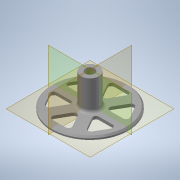
# Autodesk Inventor part: Wiel hout+spacer
Saved by Autodesk Inventor 2021 (Build 250183000, 183)
## iProperties
Manager: PJ / DCS
Company: Emmaüs Bovenbouw Aalter
Created: 2021-01-10
Part Number: Wiel hout+spacer
Material: S235
Catalog Web Link: http://emmausbovenbouw.op-weg.be/
Vendor: Emmaüsinstituut Bovenbouw Aalter
Document SubType Name: Modeling
Designer: Antho
Engineer: Declercq St.
Manufacturer: Standard
Standards Organization: Custom
Density: 7.86 g/cm^3
Appearance: Steel
Title: Algemene titel
Subject: Specifieke titel
Author: Antho
Keywords: Ruwe Ø xxxxx
Comments: Opmerking
Autodesk Inventor part; units mm, degrees
sketch "Sketch1" plane through (0, 0, 0) normal (0, 0, 1) x (1, 0, 0)
  line L0 (0, 2.8582) -> (0, -2.8582) construction
  line L1 (-5.7775, 0) -> (5.7775, 0) construction
  circle A0 centre (0, 0) radius 25.629
  circle A1 centre (0, 0) radius 4
  line L2 (0, 4) -> (0, 7)
  line L3 (0, 7) -> (0, 21)
  line L4 (0, 21) -> (5, 21)
  line L5 (5, 21) -> (8, 21)
  line L6 (8, 21) -> (0, 7)
  line L7 (0, 21) -> (-8, 21)
  line L8 (-8, 21) -> (0, 7)
  line L9 (0, -4) -> (0, -7)
  line L10 (0, -7) -> (0, -21)
  line L11 (0, -21) -> (8, -21)
  line L12 (8, -21) -> (0, -7)
  line L13 (0, -21) -> (-8, -21)
  line L14 (-8, -21) -> (0, -7)
  line L15 (0, 0) -> (2.5981, 1.5)
  line L16 (0, 0) -> (3, 0) construction
  line L17 (2.5981, 1.5) -> (3.4641, 2)
  line L18 (3.4641, 2) -> (6.0622, 3.5)
  line L19 (6.0622, 3.5) -> (18.1865, 10.5)
  line L20 (18.1865, 10.5) -> (14.1865, 17.4282)
  line L21 (14.1865, 17.4282) -> (6.0622, 3.5)
  line L22 (18.1865, 10.5) -> (22.1865, 3.5718)
  line L23 (22.1865, 3.5718) -> (6.0622, 3.5)
  line L24 (0, 0) -> (8, 0) construction
  line L25 (0, 0) -> (3.4641, -2)
  line L26 (0, 0) -> (4, 0) construction
  line L27 (3.4641, -2) -> (6.0622, -3.5)
  line L28 (6.0622, -3.5) -> (18.1865, -10.5)
  line L29 (18.1865, -10.5) -> (14.1865, -17.4282)
  line L30 (14.1865, -17.4282) -> (6.0934, -3.518)
  line L31 (18.1865, -10.5) -> (22.0919, -3.518)
  line L32 (22.0919, -3.518) -> (6.0934, -3.518)
  line L33 (0, 0) -> (-2.5981, 1.5)
  line L34 (0, 0) -> (3, 0) construction
  line L35 (-2.5981, 1.5) -> (-3.4641, 2)
  line L36 (-3.4641, 2) -> (-6.0622, 3.5)
  line L37 (-6.0622, 3.5) -> (-18.1865, 10.5)
  line L38 (-18.1865, 10.5) -> (-14.1865, 17.4282)
  line L39 (-14.1865, 17.4282) -> (-6.0622, 3.5)
  line L40 (-18.1865, 10.5) -> (-22.1865, 3.5718)
  line L41 (-22.1865, 3.5718) -> (-6.0622, 3.5)
  line L42 (0, 0) -> (-6.0622, -3.5)
  line L43 (0, 0) -> (7, 0) construction
  line L44 (-6.0622, -3.5) -> (-18.1865, -10.5)
  line L45 (-18.1865, -10.5) -> (-14.1865, -17.4282)
  line L46 (-14.1865, -17.4282) -> (-6.0622, -3.5)
  line L47 (-18.1865, -10.5) -> (-22.1865, -3.5718)
  line L48 (-22.1865, -3.5718) -> (-6.0622, -3.5)
  dimension "d0" = 51.258
  dimension "d1" = 8
  dimension "d2" = 3
  dimension "d3" = 14
  dimension "d4" = 5
  dimension "d5" = 3
  dimension "d6" = 8
  dimension "d7" = 3
  dimension "d8" = 14
  dimension "d9" = 8
  dimension "d10" = 8
  dimension "d11" = 3
  dimension "d12" = 30
  dimension "d13" = 3
  dimension "d14" = 14
  dimension "d15" = 8
  dimension "d16" = 8
  dimension "d19" = 4
  dimension "d20" = 30
  dimension "d21" = 3
  dimension "d22" = 14
  dimension "d23" = 8
  dimension "d24" = 8
  dimension "d25" = 3
  dimension "d26" = 150
  dimension "d27" = 1
  dimension "d28" = 180
  dimension "d29" = 3
  dimension "d30" = 180
  dimension "d31" = 180
  dimension "d32" = 8
  dimension "d33" = 8
  dimension "d34" = 7
  dimension "d35" = 150
  dimension "d36" = 14
  dimension "d37" = 180
  dimension "d38" = 8
  dimension "d39" = 8
  constraints: 98 end point, 12 point on line, 8 horizontal, 7 perpendicular, 4 equal length, 3 coincident, 3 collinear, 3 point on circle, 2 centre point, 2 midpoint, 2 vertical
  measures "d0" diameter of A0
  measures "d1" diameter of A1
  measures "d2" distance of L2.start L2.end
  measures "d3" distance of L2.end L3.end
  measures "d4" distance of L3.end L4.end
  measures "d5" distance of L4.end L5.end
  measures "d6" distance of L3.end L7.end
  measures "d7" distance of L9.start L9.end
  measures "d8" distance of L9.end L10.end
  measures "d9" distance of L10.end L11.end
  measures "d10" distance of L10.end L13.end
  measures "d11" distance of L15.start L15.end
  measures "d12" angle of L16 L15
  measures "d13" distance of L17.end L18.end
  measures "d14" distance of L18.end L19.end
  measures "d15" distance of L19.end L20.end
  measures "d16" distance of L19.end L22.end
  measures "d19" distance of L15.start L25.end
  measures "d20" angle of L25 L26
  measures "d21" distance of L25.end L27.end
  measures "d22" distance of L27.end L28.end
  measures "d23" distance of L28.end L29.end
  measures "d24" distance of L28.end L31.end
  measures "d25" distance of L15.start L33.end
  measures "d26" angle of L34 L33
  measures "d27" distance of L33.end L35.end
  measures "d28" angle of L35 L33
  measures "d29" distance of L35.end L36.end
  measures "d30" angle of L35 L36
  measures "d31" angle of L36 L37
  measures "d32" distance of L37.end L38.end
  measures "d33" distance of L37.end L40.end
  measures "d34" distance of L15.start L42.end
  measures "d35" angle of L42 L43
  measures "d36" distance of L42.end L44.end
  measures "d37" angle of L44 L42
  measures "d38" distance of L44.end L45.end
  measures "d39" distance of L44.end L47.end
extrude "Extrusion1" add sketch "Sketch1" along normal blind 2
fillet "Fillet1" radius 2 18 edges at (14.1865, 17.4282, 1) (22.1865, 3.5718, 1) (6.0622, 3.5, 1) (22.0919, -3.518, 1) (14.1865, -17.4282, 1) (6.0934, -3.518, 1) (0, 7, 1) (-8, 21, 1) (8, 21, 1) (-6.0622, 3.5, 1) (-22.1865, 3.5718, 1) (-14.1865, 17.4282, 1) (-6.0622, -3.5, 1) (-14.1865, -17.4282, 1) (-22.1865, -3.5718, 1) (-8, -21, 1) (0, -7, 1) (8, -21, 1)
sketch "Sketch2" plane through (0, 0, 2) normal (0, 0, 1) x (1, 0, 0)
  circle A0 centre (0, 0) radius 3.05
  circle A1 centre (0, 0) radius 5
  dimension "d43" = 6.1
  dimension "d49" = 10
  constraints: 2 centre point, 2 coincident
  measures "d43" diameter of A0
  measures "d49" diameter of A1
extrude "Extrusion2" add sketch "Sketch2" against normal blind 2
chamfer "Chamfer1" distance 1 angle 45 1 edges at (-25.629, 0, 2)
sketch "Sketch4" plane through (0, 0, 2) normal (0, 0, 1) x (1, 0, 0)
  circle A0 centre (0, 0) radius 3.05
  circle A1 centre (0, 0) radius 6
  dimension "d54" = 6.1
  dimension "d55" = 12
  constraints: 2 centre point, 2 coincident
  measures "d54" diameter of A0
  measures "d55" diameter of A1
extrude "Extrusion4" add sketch "Sketch4" along normal blind 20
fillet "Fillet2" radius 2 1 edges at (-6, 0, 2)
body "Solid1"
